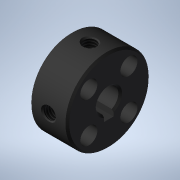
# Autodesk Inventor part: SC  0610CKP4
Saved by Autodesk Inventor 2021 (Build 250183000, 183)
## iProperties
Created: 2025-08-06
Part Number: SC  0610CKP4
Material: Generic
Catalog Web Link: www.cadenas.de
Description: Standard Set Collars-4 holes For fixation with key geoove type-part-Standard Set Collars-4 holes For fixation with key geoove type-part
Vendor: IWATA
Document SubType Name: Modeling
Designer: psAdmin
Manufacturer: IWATA
Mass: 2.69428 g
Surface Area: 21.2219 cm^2
Volume: 2.69428 cm^3
Density: 1 g/cm^3
Appearance: PSOLRGB-175-175-175
Category: PARTsolutions
Company: IWATA
Title: SC  0610CKP4
Author: Cadenas PARTsolutions
Comments: Standard Set Collars-4 holes For fixation with key geoove type-part
PSOL_IDENT_0: {$CADENAS_DATA/23d-libs/iwata/standard_set_collars/with_key_groove_type/with_key_groove_type_and_4_h
PSOL_IDENT_1: oles/parts/ssetc_4hffwkgt_p.prj},225 {VTYP=3D},{NB=SC  0610CKP4},{LINA=SC  0610CKP4},{NN=Standard Se
PSOL_IDENT_2: t Collars-4 holes For fixation with key geoove type-part},{DATE=13.01.2022 05:15:22},{GEOMDATE=02.07
PSOL_IDENT_3: .2007 00:00:00},{VERSION=},{LINEID=20},{WBVAR=},{WBNUMERIC=}  {NB=SC  0610CKP4},{LINA=SC  0610CKP4},
PSOL_IDENT_4: {KT=DUMMY},{MAT=Steel,Black},{B=6},{L=10},{D=22},{F=2.5},{G=7.2},{S=4.5},{PCD=15},{M=M4 x 4},{ORDERN
PSOL_IDENT_5: UMBER=SC  0610CKP4},{SMX=C},{C=0.5},{NDM=4},{KDM=3.242},{H=4}
NB: SC  0610CKP4
NN: Standard Set Collars-4 holes For fixation with key geoove type-part
NT: Standard Set Collars-4 holes For fixation with key geoove type-part
NBSYN: $ORDERNUMBER.
LINA: SC  0610CKP4
CATALOG: IWATA MFG. CO., LTD
MAT: Steel,Black
B: 6
L: 10
D: 22
F: 2.5
G: 7.2
S: 4.5
PCD: 15
SMX: C
C: 0.5
NDM: 4
KDM: 3.242
H: 4
SUPPLIER: IWATA
ARTICLENO: SC  0610CKP4
BOMINFO: SC  0610CKP4
CREATOR: CADENAS GmbH
Autodesk Inventor part; units mm, degrees
sketch "Sketch_1" plane through (0, 0, 0) normal (0, 0, 1) x (1, 0, 0)
  line L0 (10, 0) -> (0, 0)
  line L1 (0, 3.5) -> (0.5, 3)
  line L2 (0.5, 3) -> (9.5, 3)
  line L3 (9.5, 3) -> (10, 3.5)
  line L4 (10, 3.5) -> (10, 10.5)
  line L5 (10, 10.5) -> (9.5, 11)
  line L6 (9.5, 11) -> (0.5, 11)
  line L7 (0.5, 11) -> (0, 10.5)
  line L8 (0, 10.5) -> (0, 3.5)
  constraints: 18 end point
revolve "Revolution1" add sketch "Sketch_1" angle 360 about axis through (10, 0, 0) along (1, 0, 0)
sketch "Sketch_4" plane through (5, 0, 0) normal (1, 0, 0) x (0, 0, -1)
  line L0 (0, 1.5) -> (0, 11)
  line L1 (0, 11) -> (2, 11)
  line L2 (2, 11) -> (1.621, 10.621)
  line L3 (1.621, 10.621) -> (1.621, 1.5)
  line L4 (1.621, 1.5) -> (0, 1.5)
  line L5 (0, 1.5) -> (0, 11)
  constraints: 12 end point
revolve "Revolution2" cut sketch "Sketch_4" angle 360 about axis through (5, 1.5, 0) along (0, -1, 0)
thread "Thread1" size "M4x0.7" class "6H" standard "ISO Metric profile" length 7.621
sketch "Sketch_3" plane through (5, 0, 0) normal (1, 0, 0) x (0, 0, -1)
  line L0 (-1.5, 0) -> (-11, 0)
  line L1 (-11, 0) -> (-11, 2)
  line L2 (-11, 2) -> (-10.621, 1.621)
  line L3 (-10.621, 1.621) -> (-1.5, 1.621)
  line L4 (-1.5, 1.621) -> (-1.5, 0)
  line L5 (-1.5, 0) -> (-11, 0)
  constraints: 12 end point
revolve "Revolution3" cut sketch "Sketch_3" angle 360 about axis through (5, 0, 1.5) along (0, 0, -1)
thread "Thread2" size "M4x0.7" class "6H" standard "ISO Metric profile" length 7.621
sketch "Sketch_2" plane through (5, 0, 0) normal (1, 0, 0) x (0, 0, -1)
  line L0 (-1.25, 0) -> (-1.25, -4.2)
  line L1 (-1.25, -4.2) -> (1.25, -4.2)
  line L2 (1.25, -4.2) -> (1.25, 0)
  line L3 (1.25, 0) -> (-1.25, 0)
  constraints: 8 end point
extrude "Extrusion1" cut sketch "Sketch_2" along normal mid plane 10
sketch "Sketch_6" plane through (5, 0, 0) normal (1, 0, 0) x (0, 0, -1)
  circle A0 centre (5.3033, 5.3033) radius 2.25
  constraints: 1 centre point
extrude "Extrusion2" cut sketch "Sketch_6" along normal mid plane 10
sketch "Sketch_7" plane through (5, 0, 0) normal (1, 0, 0) x (0, 0, -1)
  circle A0 centre (-5.3033, 5.3033) radius 2.25
  constraints: 1 centre point
extrude "Extrusion3" cut sketch "Sketch_7" along normal mid plane 10
sketch "Sketch_8" plane through (5, 0, 0) normal (1, 0, 0) x (0, 0, -1)
  circle A0 centre (-5.3033, -5.3033) radius 2.25
  constraints: 1 centre point
extrude "Extrusion4" cut sketch "Sketch_8" along normal mid plane 10
sketch "Sketch_9" plane through (5, 0, 0) normal (1, 0, 0) x (0, 0, -1)
  circle A0 centre (5.3033, -5.3033) radius 2.25
  constraints: 1 centre point
extrude "Extrusion5" cut sketch "Sketch_9" along normal mid plane 10
ref_plane "part_XY" through (0, 0, 0) normal (-1, 0, 0) x (0, 0, -1)
ref_plane "part_YZ" through (0, 0, 0) normal (0, 0, -1) x (0, -1, 0)
ref_plane "part_ZX" through (0, 0, 0) normal (0, -1, 0) x (-1, 0, 0)
body "Solid1"
